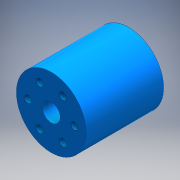
# Autodesk Inventor part: smallSprocketHolder
Saved by Autodesk Inventor 2016 (Build 200138000, 138)
## iProperties
Created: 2016-05-21
Part Number: smallSprocketHolder
Material: ABS Plastic
Document SubType Name: Modeling
Designer: Henrik Samuelsson
Density: 1.06 g/cm^3
Appearance: Smooth - White
Author: Henrik Samuelsson
Autodesk Inventor part; units mm, degrees
ref_plane "YZ Plane" through (0, 0, 0) normal (1, 0, 0) x (0, 1, 0)
ref_plane "XZ Plane" through (0, 0, 0) normal (0, 1, 0) x (-1, 0, 0)
ref_plane "XY Plane" through (0, 0, 0) normal (0, 0, 1) x (1, 0, 0)
sketch "Sketch2" plane through (0, 0, 0) normal (0, 1, 0) x (-1, 0, 0)
  circle A0 centre (0, 0) radius 3.1
  circle A1 centre (0, 0) radius 12
  circle A2 centre (8, 0) radius 1.23
  circle A3 centre (4, 6.9282) radius 1.23
  circle A4 centre (-4, 6.9282) radius 1.23
  circle A5 centre (-8, 0) radius 1.23
  circle A6 centre (-4, -6.9282) radius 1.23
  circle A7 centre (4, -6.9282) radius 1.23
  dimension "d12" = 6.2
  dimension "d14" = 24
  dimension "d15" = 2.46
  dimension "d16" = 0
  dimension "d17" = 8
  dimension "d20" = 360
  constraints: 8 centre point, 1 coincident, 1 concentric, 13 other
  measures "d12" diameter of A0
  measures "d14" diameter of A1
  measures "d15" diameter of A2
  measures "d16" vertical distance of point (0, 0) A2.centre
  measures "d17" distance of point (0, 0) A2.centre
extrude "Extrusion2" add sketch "Sketch2" along normal blind 26.68
body "Solid2"
